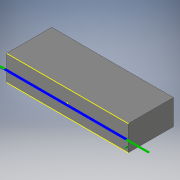
# Autodesk Inventor part: Facing Blank
Saved by Autodesk Inventor 2018.3 (Build 223284000, 284)
## iProperties
Created: 2018-11-09
Part Number: Facing Blank
Material: 4140
Document SubType Name: Sheet Metal
Designer: machinetools
Stock Number: =<Thickness> - <Material>
Density: 7.86109 g/cm^3
Sheet Metal Rule: Default
Appearance: 4140
Thickness: 0.120 in
Author: machinetools
Autodesk Inventor part; units mm, degrees
ref_plane "Right" through (0, 0, 0) normal (1, 0, 0) x (0, 1, 0)
ref_plane "Top" through (0, 0, 0) normal (0, 1, 0) x (-1, 0, 0)
ref_plane "Front" through (0, 0, 0) normal (0, 0, 1) x (1, 0, 0)
sketch "Sketch1" plane through (0, 0, 0) normal (0, 0, 1) x (1, 0, 0)
  line L0 (-107.95, 22.4282) -> (107.95, 22.4282)
  line L1 (107.95, 22.4282) -> (107.95, -22.4282)
  line L2 (107.95, -22.4282) -> (-107.95, -22.4282)
  line L3 (-107.95, -22.4282) -> (-107.95, 22.4282)
  line L4 (-107.95, 22.4282) -> (107.95, -22.4282) construction
  line L5 (107.95, 22.4282) -> (-107.95, -22.4282) construction
  point P0 (0, 0)
  dimension "d0" = 215.9
  dimension "d1" = 44.8564
  constraints: 12 end point, 2 midpoint, 2 parallel, 1 horizontal, 1 perpendicular
  measures "d0" distance of L1.end L2.end
  measures "d1" distance of L0.end L1.end
extrude "Extrusion1" add sketch "Sketch1" along normal blind 80.01
sketch "Sketch2" plane through (0, 0, 80.01) normal (0, 0, 1) x (1, 0, 0)
  line L0 (-107.95, -22.4282) -> (107.95, -22.4282) projected
  line L1 (107.95, 22.4282) -> (-107.95, 22.4282) projected
  point P0 (0, 0)
equation "\"BendRadius\" = Thickness"
equation "\"BendReliefWidth\" = 0.5 * Thickness"
equation "\"BendReliefDepth\" = 0.5 * Thickness"
equation "\"CornerReliefSize\" = 4 * Thickness"
equation "\"MinimumRemnant\" = 2 * Thickness"
equation "\"TransitionRadius\" = BendRadius"
equation "\"JacobiRadiusSize\" = BendRadius"
equation "\"Thickness\" = 3.048"
body "Solid1"
